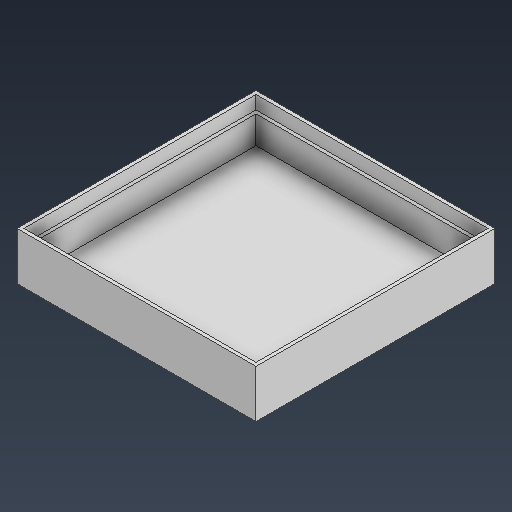
# Autodesk Inventor part: Box
Saved by Autodesk Inventor 2025.3 (Build 293356000, 356)
## iProperties
Created: 2025-09-15
Part Number: Box
Material: Generic
Document SubType Name: Modeling
Designer: tolga
Density: 1 g/cm^3
Appearance: Default
Author: tolga
Autodesk Inventor part; units mm, degrees
ref_plane "YZ Plane" through (0, 0, 0) normal (1, 0, 0) x (0, 1, 0)
ref_plane "XZ Plane" through (0, 0, 0) normal (0, 1, 0) x (-1, 0, 0)
ref_plane "XY Plane" through (0, 0, 0) normal (0, 0, 1) x (1, 0, 0)
sketch "Sketch1" plane through (0, 0, 0) normal (0, 1, 0) x (-1, 0, 0)
  line L0 (0, 0) -> (175, 0)
  line L1 (175, 0) -> (175, -175)
  line L2 (175, -175) -> (0, -175)
  line L3 (0, -175) -> (0, 0)
  dimension "d0" = 175
  dimension "d1" = 175
  constraints: 8 end point, 2 parallel, 1 horizontal, 1 perpendicular
  measures "d0" distance of L1.end L2.end
  measures "d1" distance of L0.end L1.end
extrude "Extrusion1" add sketch "Sketch1" along normal blind 5
sketch "Sketch2" plane through (0, 5, 0) normal (0, 1, 0) x (1, 0, 0)
  line L0 (0, 175) -> (-175, 175) projected
  line L1 (-175, 175) -> (-175, 0) projected
  line L2 (-175, 0) -> (0, 0) projected
  line L3 (0, 0) -> (0, 175) projected
  line L4 (-5, 170) -> (-170, 170)
  line L5 (-170, 170) -> (-170, 5)
  line L6 (-170, 5) -> (-5, 5)
  line L7 (-5, 5) -> (-5, 170)
  dimension "d4" = 5
  constraints: 8 end point, 3 other
  measures "d4" distance between parallel lines of L3 L7
extrude "Extrusion2" add sketch "Sketch2" along normal blind 30
sketch "Sketch3" plane through (0, 35, 0) normal (0, 1, 0) x (1, 0, 0)
  line L0 (-175, 175) -> (-175, 0) projected
  line L1 (-175, 0) -> (0, 0) projected
  line L2 (0, 0) -> (0, 175) projected
  line L3 (0, 175) -> (-175, 175) projected
  line L4 (-5, 170) -> (-5, 5) projected
  line L5 (-5, 5) -> (-170, 5) projected
  line L6 (-170, 5) -> (-170, 170) projected
  line L7 (-170, 170) -> (-5, 170) projected
  line L8 (-2.5, 2.5) -> (-2.5, 172.5)
  line L9 (-2.5, 172.5) -> (-172.5, 172.5)
  line L10 (-172.5, 172.5) -> (-172.5, 2.5)
  line L11 (-172.5, 2.5) -> (-2.5, 2.5)
  dimension "d7" = 2.5
  constraints: 8 end point, 3 other
  measures "d7" distance between parallel lines of L4 L8
extrude "Extrusion3" cut sketch "Sketch3" against normal blind 9.8 contours L11 L10 L9 L8
sketch "Sketch4" plane through (0, 0, 0) normal (0, -1, 0) x (1, 0, 0)
  line L0 (0, -175) -> (-175, -175) construction
  line L1 (0, 0) -> (0, -175) construction
  line L2 (-175, 0) -> (0, 0) construction
  line L3 (-175, -175) -> (-175, 0) construction
  circle A0 centre (-165, -10) radius 3.175
  circle A1 centre (-165, -165) radius 3.175
  circle A2 centre (-10, -165) radius 3.175
  circle A3 centre (-10, -10) radius 3.175
  dimension "d10" = 6.35
  dimension "d11" = 10
  dimension "d12" = 10
  dimension "d13" = 6.35
  dimension "d14" = 6.35
  dimension "d15" = 6.35
  dimension "d16" = 10
  dimension "d17" = 10
  constraints: 4 centre point, 2 horizontal alignment, 2 vertical alignment
  measures "d10" diameter of A0
  measures "d11" distance from line of L3 A0.centre
  measures "d12" distance from line of L2 A0.centre
  measures "d13" diameter of A1
  measures "d14" diameter of A2
  measures "d15" diameter of A3
  measures "d16" distance from line of L0 A2.centre
  measures "d17" distance from line of L1 A2.centre
extrude "Extrusion4" cut sketch "Sketch4" against normal blind 3.8
equation "\"d12\" = d11"
equation "\"d16\" = d11"
equation "\"d17\" = d11"
body "Solid1"
